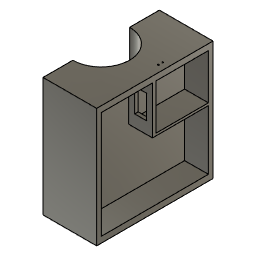
Sensor Package v1 (Autodesk Fusion 360 design; units mm, degrees)
Autodesk Fusion 360 part; units mm, degrees
note: some values were not read from the file. Set by a fixed rule: which sketch regions a step uses.
sketch "Sketch1" plane through (0, 0, 0) normal (0, 0, 1) x (1, 0, 0)
  arc A0 (0.1047, -30.3528) -> (-0.0415, 30.353) centre (0, 0) ccw
  line L0 (-0.0415, 30.353) -> (-0.0415, 62.103)
  line L1 (0.1047, -30.3528) -> (0.1047, -62.1028)
  line L2 (-0.0415, 62.103) -> (57.1085, 62.103)
  line L3 (0.1047, -62.1028) -> (57.2547, -62.1028)
  line L4 (57.1085, 62.103) -> (57.2547, -62.1028)
  dimension "d1" = 60.706
  dimension "d10" = 31.75
  dimension "d12" = 57.15
  constraint coincident A0.centre origin
  constraint vertical L0
  constraint vertical L1
  constraint perpendicular L0 L2
  constraint perpendicular L1 L3
  constraint equal L2 L3
  constraint equal L0 L1
  measures "d1" diameter of A0
  measures "d10" distance of A0.end L0.end
  measures "d12" distance of L0.end L2.end
extrude "Extrude1" add sketch "Sketch1" along normal mid plane 127
sketch "Sketch4" plane through (57.1815, 0.0673, 0) normal (0.999999, 0.001177, 0) x (-0.001177, 0.999999, 0)
  line L0 (62.0357, -63.5) -> (62.0357, 63.5)
  line L1 (62.0357, 63.5) -> (-62.1702, 63.5)
  line L2 (-62.1702, 63.5) -> (-62.1702, -63.5)
  line L3 (-62.1702, -63.5) -> (62.0357, -63.5)
  line L4 (57.15, -57.15) -> (-57.15, -57.15)
  line L5 (-57.15, -57.15) -> (-57.15, 57.15)
  line L6 (-57.15, 57.15) -> (-2.54, 57.15)
  line L7 (57.15, 6.35) -> (57.15, -57.15)
  line L8 (57.15, -57.15) -> (-57.15, 57.15) construction
  line L9 (-57.15, -57.15) -> (57.15, 57.15) construction
  line L10 (-2.54, 57.15) -> (-2.54, 6.35)
  line L11 (-2.54, 6.35) -> (57.15, 6.35)
  dimension "d21" = 114.3
  dimension "d22" = 114.3
  dimension "d35" = 59.69
  dimension "d36" = 50.8
  constraint horizontal L4
  constraint perpendicular L4 L5
  constraint parallel L4 L6
  constraint parallel L5 L7
  constraint vertical L10
  constraint horizontal L11
  measures "d21" distance of L5.end L9.end
  measures "d22" distance of L4.end L5.end
  measures "d35" distance of L9.end L6.end
  measures "d36" distance of L9.end L7.start
extrude "Extrude3" cut sketch "Sketch4" against normal blind 25.4 contours L4 L5 L6 L7 L10 L11
sketch "Sketch6" plane through (57.1815, 0.0673, 0) normal (0.999999, 0.001177, 0) x (-0.001177, 0.999999, 0)
  line L0 (-57.15, 57.15) -> (-2.54, 57.15)
  line L1 (-2.54, 57.15) -> (-2.54, 6.35)
  line L2 (-2.54, 6.35) -> (57.15, 6.35)
  line L3 (57.15, 6.35) -> (57.15, -57.15)
  line L4 (57.15, -57.15) -> (-57.15, -57.15)
  line L5 (-57.15, -57.15) -> (-57.15, 57.15)
  line L6 (62.0357, -63.5) -> (62.0357, 63.5)
  line L7 (62.0357, 63.5) -> (-62.1702, 63.5)
  line L8 (-62.1702, 63.5) -> (-62.1702, -63.5)
  line L9 (-62.1702, -63.5) -> (62.0357, -63.5)
  line L10 (1.27, 57.15) -> (57.15, 57.15)
  line L11 (57.15, 57.15) -> (57.15, 8.89)
  line L12 (57.15, 8.89) -> (1.27, 8.89)
  line L13 (1.27, 8.89) -> (1.27, 57.15)
  dimension "d37" = 55.88
  dimension "d38" = 48.26
  constraint horizontal L10
  constraint vertical L11
  constraint horizontal L12
  constraint vertical L13
  constraint collinear L3 L11
  measures "d37" distance of L10.start L10.end
  measures "d38" distance of L10.start L12.end
extrude "Extrude5" cut sketch "Sketch6" against normal blind 25.4 contours L10 L11 L12 L13
sketch "Sketch8" plane through (0, 0, 63.5) normal (0, 0, 1) x (-1, 0, 0)
  line L0 (-0.1047, 30.3528) -> (-0.1047, 62.1028)
  line L1 (-0.1047, 62.1028) -> (-57.2547, 62.1028)
  line L2 (-57.2547, 62.1028) -> (-57.1085, -62.103)
  line L3 (-57.1085, -62.103) -> (0.0415, -62.103)
  line L4 (0.0415, -62.103) -> (0.0415, -30.353)
  arc A0 (-0.1047, 30.3528) -> (0.0415, -30.353) centre (0, 0) ccw
  circle A1 centre (-49.9987, -11.1079) radius 0.8001
  circle A2 centre (-49.9987, -15.6799) radius 0.8001
  line L5 (-57.18, -1.3373) -> (-31.7801, -1.3074)
  dimension "d45" = 1.6002
  dimension "d46" = 4.572
  dimension "d47" = 9.779
  constraint equal A1 A2
  measures "d45" diameter of A1
  measures "d46" distance of A1.centre A2.centre
  measures "d47" distance of A1.centre L5
extrude "Extrude6" cut sketch "Sketch8" against normal up to surface (6.35 mm away) contours A1 | A2
sketch "Sketch9" plane through (0.003, -2.54, 0) normal (0.001177, -0.999999, 0) x (0.999999, 0.001177, 0)
  line L0 (57.1816, 6.35) -> (57.1816, 57.15)
  line L1 (57.1816, 57.15) -> (31.7816, 57.15)
  line L2 (31.7816, 57.15) -> (31.7816, 6.35)
  line L3 (31.7816, 6.35) -> (57.1816, 6.35)
  line L4 (50.8316, 44.45) -> (38.1316, 44.45)
  line L5 (38.1316, 44.45) -> (38.1316, 19.05)
  line L6 (38.1316, 19.05) -> (50.8316, 19.05)
  line L7 (50.8316, 19.05) -> (50.8316, 44.45)
  dimension "d50" = 12.7
  dimension "d51" = 25.4
  dimension "d52" = 12.7
  dimension "d54" = 6.35
  constraint horizontal L4
  constraint vertical L5
  constraint horizontal L6
  constraint vertical L7
  measures "d50" distance of L4.start L4.end
  measures "d51" distance of L4.start L6.end
  measures "d52" distance of L3 L6
  measures "d54" distance of L0 L7
extrude "Extrude7" cut sketch "Sketch9" against normal up to surface (3.81 mm away) contours L4 L5 L6 L7
